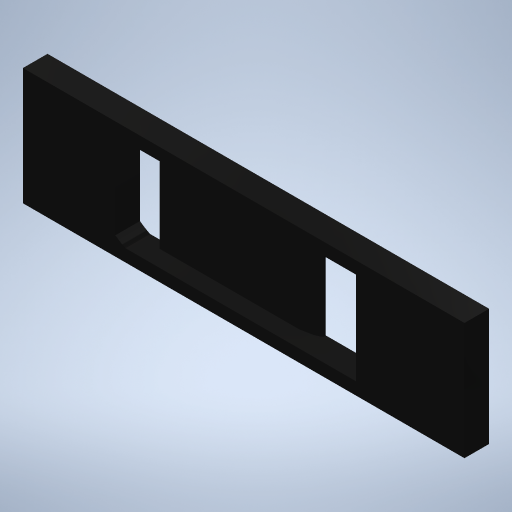
# Autodesk Inventor part: backplate-0
Saved by Autodesk Inventor 2023 (Build 270158030, 158C)
## iProperties
Created: 2024-09-24
Part Number: backplate-0
Material: Generic
Document SubType Name: Modeling
Designer: Imogen Heard
Density: 1 g/cm^3
Appearance: Glossy - Black
Author: Imogen Heard
Autodesk Inventor part; units mm, degrees
ref_plane "YZ Plane" through (0, 0, 0) normal (1, 0, 0) x (0, 1, 0)
ref_plane "XZ Plane" through (0, 0, 0) normal (0, 1, 0) x (-1, 0, 0)
ref_plane "XY Plane" through (0, 0, 0) normal (0, 0, 1) x (1, 0, 0)
ref_plane "Work Plane1" through (2.7698, 1, -3.5) normal (0, 0, 1) x (1, 0, 0)
sketch "Sketch1" plane through (0, 0, 0) normal (0, 0, 1) x (1, 0, 0)
  line L0 (34.0626, 1) -> (0, 1) projected
  line L1 (34.0626, 14) -> (34.0626, 1) projected
  line L2 (0, 14) -> (34.0626, 14) projected
  line L3 (0, 1) -> (0, 14) projected
  arc A0 (1.6411, 15) -> (0, 14) centre (6, 6) ccw projected
  line L4 (0, 14) -> (34.0626, 14) projected
  line L5 (34.0626, 15) -> (34.0626, 14) projected
  line L6 (34.0626, 15) -> (1.6411, 15) projected
  line L7 (1.6411, 0) -> (34.0626, 0) projected
  arc A1 (0, 1) -> (1.6411, 0) centre (6, 9) ccw projected
  line L8 (1.6411, 0) -> (34.0626, 0) projected
  line L9 (34.0626, 0) -> (34.0626, 1) projected
  line L10 (34.0626, 1) -> (0, 1) projected
  line L11 (-15, 17) -> (56.6619, 17)
  line L12 (56.6619, 17) -> (56.6619, -2)
  line L13 (56.6619, -2) -> (-15, -2)
  line L14 (-15, -2) -> (-15, 17)
  line L15 (70.331, 1) -> (64.4317, 1) projected
  arc A2 (70.331, 1) -> (70.331, 14) centre (70.331, 7.5) ccw projected
  line L16 (64.4317, 14) -> (70.331, 14) projected
  line L17 (64.4317, 1) -> (64.4317, 14) projected
  arc A3 (70.331, 0) -> (70.331, 15) centre (70.331, 7.5) ccw projected
  line L18 (-22.7698, 1) -> (-28.669, 1) projected
  line L19 (-22.7698, 14) -> (-22.7698, 1) projected
  line L20 (-28.669, 14) -> (-22.7698, 14) projected
  arc A4 (-28.669, 14) -> (-28.669, 1) centre (-28.669, 7.5) ccw projected
  arc A5 (-28.669, 15) -> (-28.669, 0) centre (-28.669, 7.5) ccw projected
  line L21 (34.0626, 1) -> (41.6619, 1) projected
  line L22 (41.6619, 14) -> (34.0626, 14) projected
  line L23 (34.0626, 15) -> (41.004, 15) projected
  line L24 (41.004, 0) -> (34.0626, 0) projected
  line L25 (41.6619, 1) -> (41.6619, 14) projected
  line L26 (34.0626, 15) -> (39.0626, 15)
  line L27 (39.0626, 15) -> (39.0626, 0)
  line L28 (39.0626, 0) -> (34.0626, 0)
  line L29 (34.0626, 0) -> (34.0626, 15)
  point P0 (0, 0)
  point P1 (20.831, 17)
  point P2 (-30.669, 13.6847)
  point P3 (-30.669, 1.3153)
  point P4 (39.0626, 14)
  point P5 (39.0626, 1)
  point P6 (39.0626, 0)
  dimension "d0" = 2
  dimension "d11" = 5
  dimension "d36" = 15
  dimension "d37" = 2
  dimension "d38" = 15
  constraints: 16 end point, 4 parallel, 2 horizontal, 2 perpendicular, 1 midpoint
  measures "d0" distance from line of point (20.831, 17) L6
  measures "d11" distance between parallel lines of L27 L9
  measures "d36" distance between parallel lines of L14 L3
  measures "d37" distance between parallel lines of L13 L7
  measures "d38" distance between parallel lines of L25 L12
extrude "Extrusion1" add sketch "Sketch1" against normal up to surface (3.5 mm away) contours L27 L22 L25 L21 | L11 L12 L13 L14
sketch "Sketch2" plane through (1.6411, 0, 0) normal (0, 1, 0) x (1, 0, 0)
  arc A0 (32.4215, 0) -> (40.0208, 3.5) centre (32.4215, 10) ccw projected
  line L0 (32.4215, 0) -> (-1.6411, 0) projected
  arc A1 (4.3589, 2) -> (0, 1) centre (4.3589, -8) ccw projected
  line L1 (1.1287, 3.5) -> (30.0208, 3.5) projected
  line L2 (30.0208, 2) -> (4.3589, 2) projected
  line L3 (2.8589, 3.5) -> (28.5208, 3.5)
  line L4 (28.5208, 3.5) -> (28.5208, 2.2)
  line L5 (28.5208, 2.2) -> (2.8589, 2.2)
  line L6 (2.8589, 2.2) -> (2.8589, 3.5)
  line L7 (30.0208, 4.5) -> (30.0208, 2) projected
  point P0 (32.4215, 3)
  dimension "d6" = 1.5
  dimension "d7" = 0.2
  dimension "d8" = 1.5
  constraints: 8 end point, 2 parallel, 1 horizontal, 1 horizontal alignment, 1 perpendicular
  measures "d6" distance between parallel lines of L4 L7
  measures "d7" distance between parallel lines of L2 L5
  measures "d8" distance from line of L2.end L6
extrude "Extrusion2" add sketch "Sketch2" along normal up to surface (15 mm away)
chamfer "Chamfer1" distance 3.5 angle 45 1 edges at (39.0626, 7.5, -3.5)
chamfer "Chamfer4" distance 1 angle 45 1 edges at (30.1619, 7.5, -2.2)
chamfer "Chamfer5" distance 1 angle 45 1 edges at (29.1619, 7.5, -2.2)
chamfer "Chamfer6" distance 1 angle 45 1 edges at (28.1619, 7.5, -2.2)
sketch "Sketch6" plane through (0, 0, 0) normal (0, 0, 1) x (1, 0, 0)
  line L0 (-15, -2) -> (56.6619, -2) projected
  line L1 (56.6619, -2) -> (56.6619, 17) projected
  line L2 (56.6619, 17) -> (-15, 17) projected
  line L3 (-15, 17) -> (-15, -2) projected
  arc A0 (0, 1) -> (1.6411, 0) centre (6, 9) ccw projected
  line L4 (0, 1) -> (0, 14) projected
  arc A1 (1.6411, 15) -> (0, 14) centre (6, 6) ccw projected
  line L5 (1.6411, 15) -> (39.0626, 15) projected
  line L6 (39.0626, 15) -> (39.0626, 0) projected
  line L7 (39.0626, 0) -> (1.6411, 0) projected
  point P0 (0, 0)
extrude "Extrusion5" add sketch "Sketch6" along normal blind 0.5
sketch "Sketch3" plane through (-10, -5, -3.5) normal (0, 0, -1) x (-1, 0, 0)
  circle A0 centre (-3, -212) radius 1.55
  circle A1 centre (-3, 22) radius 1.55
  circle A2 centre (-87.331, -212) radius 1.55
  circle A3 centre (-87.331, 22) radius 1.55
  line L0 (-95.331, 18) -> (-95.331, -208) projected
  line L1 (-7, 30) -> (-83.331, 30) projected
  line L2 (5, -208) -> (5, 18) projected
  line L3 (-83.331, -220) -> (-7, -220) projected
  point P0 (-10, 5)
  point P1 (5, 18)
  point P2 (20.669, 6.3153)
  dimension "d16" = 3.1
  dimension "d26" = 8
  dimension "d27" = 8
  dimension "d28" = 8
  dimension "d29" = 8
  constraints: 4 centre point, 3 equal radius, 2 horizontal alignment, 2 vertical alignment, 1 other
  measures "d16" diameter of A0
  measures "d26" distance from line of L0 A3.centre
  measures "d27" distance from line of L1 A3.centre
  measures "d29" distance from line of L3 A0.centre
sketch "Sketch4" plane through (0, 0, 0) normal (0, 0, 1) x (1, 0, 0)
  circle A0 centre (77.331, 17) radius 1.55 projected
  circle A1 centre (77.331, -217) radius 1.55 projected
  circle A2 centre (-7, 17) radius 1.55 projected
  circle A3 centre (-7, -217) radius 1.55 projected
  arc A4 (-3, 25) -> (-15, 13) centre (-3, 13) ccw projected
  line L0 (-15, 13) -> (-15, -213) projected
  arc A5 (-15, -213) -> (-3, -225) centre (-3, -213) ccw projected
  line L1 (-3, -225) -> (73.331, -225) projected
  arc A6 (73.331, -225) -> (85.331, -213) centre (73.331, -213) ccw projected
  line L2 (85.331, -213) -> (85.331, 13) projected
  arc A7 (85.331, 13) -> (73.331, 25) centre (73.331, 13) ccw projected
  line L3 (73.331, 25) -> (-3, 25) projected
  line L4 (39.0626, 0) -> (1.6411, 0) projected
  arc A8 (0, 1) -> (1.6411, 0) centre (6, 9) ccw projected
  line L5 (0, 1) -> (0, 14) projected
  arc A9 (1.6411, 15) -> (0, 14) centre (6, 6) ccw projected
  line L6 (1.6411, 15) -> (39.0626, 15) projected
  line L7 (39.0626, 15) -> (39.0626, 0) projected
